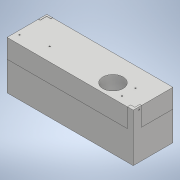
# Autodesk Inventor part: 2руб
Saved by Autodesk Inventor 2020 (Build 240168000, 168)
## iProperties
Created: 2020-02-01
Part Number: 2руб
Material: Типовые
Document SubType Name: Modeling
Designer: Css38
Density: 1 g/cm^3
Appearance: По умолчанию
Author: Css38
Autodesk Inventor part; units mm, degrees
ref_plane "YZ Plane" through (0, 0, 0) normal (1, 0, 0) x (0, 1, 0)
ref_plane "XZ Plane" through (0, 0, 0) normal (0, 1, 0) x (-1, 0, 0)
sketch "Эскиз1" plane through (0, 0, 0) normal (0, 0, 1) x (1, 0, 0)
  line L0 (-76.25, 24) -> (76.25, 24)
  line L1 (76.25, 24) -> (76.25, -24)
  line L2 (76.25, -24) -> (-76.25, -24)
  line L3 (-76.25, -24) -> (-76.25, 24)
  line L4 (-76.25, 24) -> (76.25, -24) construction
  line L5 (76.25, 24) -> (-76.25, -24) construction
  point P0 (0, 0)
  point P1 (0, 0)
  dimension "d35" = 152.5
  dimension "d36" = 48
  constraints: 12 end point, 2 parallel, 1 coincident, 1 horizontal, 1 midpoint, 1 perpendicular
  measures "d35" distance of L1.end L2.end
  measures "d36" distance of L2.end L0.start
extrude "Выдавливание1" add sketch "Эскиз1" along normal blind 30
sketch "Эскиз2" plane through (0, 0, 30) normal (0, 0, 1) x (1, 0, 0)
  line L0 (76.25, 24) -> (76.25, -24) construction
  line L1 (76.25, -24) -> (-76.25, -24) construction
  line L2 (-76.25, -24) -> (-76.25, 24) construction
  line L3 (-76.25, 24) -> (76.25, 24) construction
  line L4 (74.25, -20) -> (49.25, -20)
  line L5 (49.25, -20) -> (49.25, 5)
  line L6 (49.25, 5) -> (74.25, 5)
  line L7 (74.25, 5) -> (74.25, -20)
  point P0 (0, 0)
  dimension "d40" = 25
  dimension "d143" = 2
  dimension "d144" = 4
  constraints: 8 end point, 2 parallel, 2 perpendicular, 1 horizontal
  measures "d40" distance of L5.end L6.end
  measures "d143" distance between parallel lines of L0 L7
  measures "d144" distance between parallel lines of L1 L4
extrude "Выдавливание2" cut sketch "Эскиз2" against normal up to next
sketch "Эскиз3" plane through (0, 0, 30) normal (0, 0, 1) x (1, 0, 0)
  line L0 (49.25, 5) -> (49.25, -20)
  line L1 (49.25, -20) -> (74.25, -20)
  line L2 (74.25, -20) -> (74.25, 5)
  line L3 (74.25, 5) -> (49.25, 5)
  line L4 (76.25, 24) -> (76.25, -24) construction
  line L5 (76.25, -24) -> (-76.25, -24) construction
  line L6 (-76.25, 24) -> (76.25, 24) construction
  line L7 (76.25, 24) -> (-76.25, 24) projected
  line L8 (-76.25, 24) -> (76.25, 24)
  line L9 (76.25, 24) -> (76.25, -24)
  line L10 (76.25, -24) -> (-76.25, -24)
  line L11 (-76.25, 24) -> (-76.25, 22)
  line L12 (-76.25, 24) -> (-76.25, -24) construction
  line L13 (-76.25, 22) -> (1.25, 22)
  line L14 (1.25, 22) -> (1.25, 5)
  line L15 (1.25, 5) -> (21.25, 5)
  line L16 (21.25, 5) -> (21.25, -20)
  line L17 (21.25, -20) -> (-76.25, -20)
  line L18 (-76.25, -24) -> (-76.25, -20)
  line L19 (-76.25, -24) -> (76.25, -24) projected
  line L20 (76.25, -24) -> (76.25, 24) projected
  line L21 (74.25, -20) -> (49.25, -20) projected
  line L22 (49.25, -20) -> (49.25, 5) projected
  line L23 (49.25, 5) -> (74.25, 5) projected
  line L24 (74.25, 5) -> (74.25, -20) projected
  dimension "d50" = 2
  dimension "d63" = 28
  dimension "d130" = 20
  constraints: 34 end point, 13 collinear, 4 perpendicular, 2 parallel, 2 point on line
  measures "d50" distance of L6.start L11.end
  measures "d63" distance between parallel lines of L0 L16
  measures "d130" distance of L14.end L15.end
extrude "Выдавливание4" add sketch "Эскиз3" along normal blind 3
sketch "Эскиз4" plane through (0, 0, 33) normal (0, 0, 1) x (1, 0, 0)
  line L0 (49.25, 5) -> (49.25, -20) construction
  line L1 (49.25, -20) -> (74.25, -20) construction
  line L2 (74.25, -20) -> (74.25, 5) construction
  line L3 (74.25, 5) -> (49.25, 5) construction
  line L4 (76.25, 24) -> (76.25, -24) projected
  line L5 (76.25, -24) -> (-76.25, -24) projected
  line L6 (-76.25, -24) -> (-76.25, -20) projected
  line L7 (-76.25, -20) -> (21.25, -20) projected
  line L8 (21.25, -20) -> (21.25, 5) projected
  line L9 (21.25, 5) -> (1.25, 5) projected
  line L10 (1.25, 5) -> (1.25, 22) projected
  line L11 (1.25, 22) -> (-76.25, 22) projected
  line L12 (-76.25, 22) -> (-76.25, 24) projected
  line L13 (-76.25, 24) -> (76.25, 24) projected
  line L14 (21.25, -20) -> (21.25, 5) projected
  line L15 (21.25, 5) -> (49.25, 5) construction
  line L16 (49.25, 5) -> (49.25, -20) projected
  line L17 (49.25, -20) -> (21.25, -20) construction
  circle A0 centre (35.25, -7.5) radius 12.25
  line L18 (35.25, -7.5) -> (35.25, 5) construction
  line L19 (35.25, -7.5) -> (35.25, -20) construction
  line L20 (49.25, -20) -> (49.25, 5) construction
  line L21 (35.25, -7.5) -> (21.25, -7.5) construction
  line L22 (35.25, -7.5) -> (49.25, -7.5) construction
  point P0 (0, 0)
  dimension "d55" = 24.5
  constraints: 12 end point, 4 midpoint, 3 perpendicular, 2 collinear, 1 centre point, 1 point on line, 1 other
  measures "d55" diameter of A0
extrude "Выдавливание7" add sketch "Эскиз4" along normal blind 25
sketch "Эскиз6" plane through (21.25, -20, 30) normal (-1, 0, 0) x (0, 0, 1)
  line L0 (3, 0.25) -> (3, 24.75) construction
  line L1 (0, 25) -> (28, 25) projected
  line L2 (0, 0) -> (28, 0) projected
  line L3 (3, 25) -> (5.2, 25)
  line L4 (5.2, 25) -> (5.2, 0)
  line L5 (5.2, 0) -> (3, 0)
  line L6 (3, 0) -> (3, 25)
  point P0 (-30, 20)
  dimension "d66" = 2.2
  constraints: 8 end point, 2 parallel, 2 point on line, 1 collinear, 1 horizontal, 1 perpendicular
  measures "d66" distance of L4.end L5.end
extrude "Выдавливание8" cut sketch "Эскиз6" against normal up to surface (53 mm away) from surface at 0
sketch "Эскиз7" plane through (0, 0, 58) normal (0, 0, 1) x (1, 0, 0)
  line L0 (76.25, -24) -> (-76.25, -24) projected
  line L1 (-76.25, 24) -> (76.25, 24) projected
  line L2 (76.25, -24) -> (-76.25, -24)
  line L3 (-76.25, -24) -> (-76.25, 24)
  line L4 (-76.25, 24) -> (76.25, 24)
  line L5 (76.25, 24) -> (76.25, -24)
  circle A0 centre (35.25, -7.5) radius 12.25 projected
  point P0 (0, 0)
  constraints: 8 end point, 2 parallel, 1 horizontal, 1 perpendicular
extrude "Выдавливание9" add sketch "Эскиз7" against normal blind 17.15
ref_plane "РабПлоскость1" through (74.25, -20, 35.2) normal (0, 0, -1) x (-1, 0, 0)
split body "Разделение1" result two bodies by plane through (74.25, -20, 35.2) normal (0, 0, -1) first body at (-34.4167, 1.6667, 0.5)
sketch "Эскиз21" plane through (0, 0, 30) normal (0, 0, 1) x (1, 0, 0)
  line L0 (-76.25, -20) -> (21.25, -20) construction
  line L1 (21.25, -20) -> (21.25, 5) construction
  line L2 (21.25, 5) -> (1.25, 5) construction
  line L3 (1.25, 5) -> (1.25, 22) construction
  line L4 (1.25, 22) -> (-76.25, 22) construction
  line L5 (-76.25, -20) -> (-76.25, 22) construction
  line L6 (-76.25, -24) -> (-76.25, -20) construction
  line L7 (76.25, -24) -> (-76.25, -24) construction
  line L8 (76.25, 24) -> (76.25, -24) construction
  line L9 (-76.25, 24) -> (76.25, 24) construction
  line L10 (74.25, 5) -> (49.25, 5) construction
  line L11 (49.25, 5) -> (49.25, -20) construction
  line L12 (49.25, -20) -> (74.25, -20) construction
  line L13 (74.25, -20) -> (74.25, 5) construction
  line L14 (-76.25, -20) -> (-43.25, -20)
  line L15 (-43.25, -20) -> (-43.25, -7.5)
  line L16 (-43.25, -7.5) -> (-76.25, -7.5)
  line L17 (-76.25, -7.5) -> (-76.25, -20)
  line L18 (-76.25, 22) -> (-76.25, 24) projected
  point P0 (0, 0)
  dimension "d145" = 33
  dimension "d146" = 12.5
  constraints: 8 end point, 2 parallel, 1 horizontal, 1 perpendicular
  measures "d145" distance of L16.end L15.end
  measures "d146" distance of L15.end L14.end
extrude "Выдавливание26" cut sketch "Эскиз21" against normal blind 28 bodies 2
sketch "Эскиз22" plane through (0, 0, 2) normal (0, 0, 1) x (1, 0, 0)
  line L0 (-76.25, 24) -> (76.25, 24) construction
  line L1 (76.25, 24) -> (76.25, -24) construction
  line L2 (76.25, -24) -> (-76.25, -24) construction
  line L3 (-76.25, -24) -> (-76.25, -20) construction
  line L4 (-76.25, -20) -> (-76.25, -7.5) construction
  line L5 (-76.25, -7.5) -> (-76.25, 24) construction
  line L6 (-76.25, -20) -> (-43.25, -20) construction
  line L7 (-43.25, -20) -> (-43.25, -7.5) construction
  line L8 (-43.25, -7.5) -> (-76.25, -7.5) construction
  line L9 (74.25, 5) -> (49.25, 5) construction
  line L10 (49.25, 5) -> (49.25, -20) construction
  line L11 (49.25, -20) -> (74.25, -20) construction
  line L12 (74.25, -20) -> (74.25, 5) construction
  line L13 (-43.25, -7.5) -> (-47.75, -7.5)
  line L14 (-47.75, -7.5) -> (-47.75, -20)
  line L15 (-47.75, -20) -> (-43.25, -20)
  line L16 (-43.25, -20) -> (-43.25, -7.5)
  point P0 (0, 0)
  dimension "d149" = 4.5
  constraints: 8 end point, 2 parallel, 1 horizontal, 1 perpendicular, 1 point on line
  measures "d149" distance of L15.end L14.end
extrude "Выдавливание27" add sketch "Эскиз22" along normal blind 18 bodies 2
sketch "Эскиз23" plane through (0, 0, 20) normal (0, 0, 1) x (1, 0, 0)
  line L0 (-76.25, 24) -> (76.25, 24) construction
  line L1 (76.25, 24) -> (76.25, -24) construction
  line L2 (76.25, -24) -> (-76.25, -24) construction
  line L3 (-76.25, -24) -> (-76.25, -20) construction
  line L4 (-76.25, -20) -> (-47.75, -20) construction
  line L5 (-47.75, -20) -> (-47.75, -7.5) construction
  line L6 (-43.25, -7.5) -> (-47.75, -7.5) construction
  line L7 (-43.25, -20) -> (-43.25, -7.5) construction
  line L8 (-47.75, -20) -> (-43.25, -20) construction
  line L9 (-76.25, -7.5) -> (-76.25, 24) construction
  line L10 (-47.75, -7.5) -> (-76.25, -7.5) construction
  line L11 (74.25, 5) -> (49.25, 5) construction
  line L12 (49.25, 5) -> (49.25, -20) construction
  line L13 (49.25, -20) -> (74.25, -20) construction
  line L14 (74.25, -20) -> (74.25, 5) construction
  line L15 (-47.75, -20) -> (-43.25, -7.5) construction
  line L16 (-43.25, -20) -> (-47.75, -7.5) construction
  circle A0 centre (-45.5, -13.75) radius 0.75
  point P0 (0, 0)
  dimension "d152" = 1.5
  constraints: 4 end point, 1 centre point, 1 midpoint
  measures "d152" diameter of A0
extrude "Выдавливание28" cut sketch "Эскиз23" against normal blind 3 bodies 2
sketch "Эскиз24" plane through (0, 0, 30) normal (0, 0, 1) x (1, 0, 0)
  line L0 (-76.25, 24) -> (76.25, 24) construction
  line L1 (76.25, 24) -> (76.25, -24) construction
  line L2 (76.25, -24) -> (-76.25, -24) construction
  line L3 (-76.25, -24) -> (-76.25, -20) construction
  line L4 (-76.25, -20) -> (-43.25, -20) construction
  line L5 (-43.25, -20) -> (-43.25, -7.5) construction
  line L6 (-43.25, -7.5) -> (-76.25, -7.5) construction
  line L7 (-76.25, -7.5) -> (-76.25, 22) construction
  line L8 (1.25, 22) -> (-76.25, 22) construction
  line L9 (1.25, 5) -> (1.25, 22) construction
  line L10 (21.25, 5) -> (1.25, 5) construction
  line L11 (21.25, -20) -> (21.25, 5) construction
  line L12 (-43.25, -20) -> (21.25, -20) construction
  line L13 (74.25, 5) -> (49.25, 5) construction
  line L14 (49.25, 5) -> (49.25, -20) construction
  line L15 (49.25, -20) -> (74.25, -20) construction
  line L16 (74.25, -20) -> (74.25, 5) construction
  line L17 (-43.25, -7.5) -> (-43.25, -20) construction
  line L18 (-76.25, -20) -> (-76.25, -7.5) construction
  line L19 (-65.25, -13.75) -> (-48.2817, 16.8617)
  line L20 (-48.2817, 16.8617) -> (-27.533, -7.5)
  line L21 (-27.533, -7.5) -> (21.467, -7.5)
  line L22 (-76.25, 22) -> (-76.25, 24) projected
  point P0 (0, 0)
  point P1 (-43.25, -13.75)
  point P2 (49.25, -7.5)
  dimension "d155" = 11
  dimension "d156" = 49
  dimension "d157" = 35
  dimension "d161" = 32
  dimension "d162" = 61
  constraints: 6 end point, 2 midpoint, 1 horizontal, 1 horizontal alignment, 1 point on line
  measures "d155" distance from line of L18 L19.start
  measures "d156" distance of L20.end L21.end
  measures "d157" distance of L19.start L19.end
  measures "d161" distance of L19.end L20.end
  measures "d162" angle of L12 L19
sketch "Эскиз20" plane through (0, 0, 58) normal (0, 0, 1) x (1, 0, 0)
  line L0 (76.25, -24) -> (-76.25, -24) construction
  line L1 (-76.25, -24) -> (-76.25, 24) construction
  line L2 (59.5, -24) -> (-46, -24) construction
  line L3 (-46, -24) -> (-46, 8.5) construction
  line L4 (-46, 8.5) -> (59.5, 8.5) construction
  line L5 (0, -33.6) -> (0, 33.6) construction
  line L6 (59.5, 8.5) -> (59.5, -24) construction
  circle A0 centre (35.25, -7.5) radius 12.25 construction
  line L7 (-76.25, -24) -> (76.25, -24) construction
  line L8 (-76.25, -24) -> (76.25, -24) construction
  circle A1 centre (-71.25, -13.8) radius 0.5
  line L9 (-36, 8.5) -> (-36, -24) construction
  line L10 (49.5, -24) -> (49.5, 8.5) construction
  line L11 (-46, 8.5) -> (-36, -24) construction
  line L12 (-36, 8.5) -> (-46, -24) construction
  line L13 (59.5, 8.5) -> (49.5, -7.75) construction
  line L14 (49.5, -7.75) -> (59.5, -24) construction
  line L15 (49.5, -24) -> (59.5, -7.75) construction
  line L16 (59.5, -7.75) -> (49.5, 8.5) construction
  circle A2 centre (-41, -7.75) radius 0.5
  circle A3 centre (54.5, 0.375) radius 0.5
  circle A4 centre (54.5, -15.875) radius 0.5
  point P0 (0, 0)
  point P1 (-76.25, 14)
  dimension "d131" = 32.5
  dimension "d163" = 10.2
  dimension "d164" = 5
  dimension "d165" = 105.5
  dimension "d168" = 2
  dimension "d169" = 10
  dimension "d170" = 10
  dimension "d171" = 1
  constraints: 24 end point, 5 midpoint, 4 centre point, 4 point on line, 3 equal radius, 3 parallel, 3 perpendicular, 1 collinear, 1 horizontal
  measures "d131" distance of L2.end L3.end
  measures "d163" distance from line of L0 A1.centre
  measures "d164" distance from line of L1 A1.centre
  measures "d165" distance of L3.end L4.end
  measures "d168" distance edge to line of A0 L10
  measures "d169" distance between parallel lines of L6 L10
  measures "d170" distance between parallel lines of L3 L9
  measures "d171" diameter of A1
hole "Отверстие1" at (-71.25, -13.8, 58) at (-41, -7.75, 58) at (54.5, 0.375, 58) at (54.5, -15.875, 58) direction (0, 0, -1) diameter 1 depth 3 tip angle 118 countersink diameter 1.5 countersink angle 90 bodies 3
sketch "Эскиз25" plane through (0, 0, 30) normal (0, 0, 1) x (1, 0, 0)
  line L0 (-76.25, 24) -> (76.25, 24) construction
  line L1 (-76.25, 24) -> (-76.25, 14)
  line L2 (-76.25, -24) -> (-76.25, 24) construction
  line L3 (-76.25, 14) -> (-74.25, 14)
  line L4 (-76.25, -24) -> (-76.25, -20) construction
  line L5 (-76.25, -20) -> (-43.25, -20) construction
  line L6 (-43.25, -20) -> (-43.25, -7.5) construction
  line L7 (-43.25, -7.5) -> (-76.25, -7.5) construction
  line L8 (-76.25, -7.5) -> (-76.25, 22) construction
  line L9 (-76.25, 22) -> (-76.25, 24) construction
  line L10 (-76.25, 24) -> (76.25, 24) construction
  line L11 (76.25, 24) -> (76.25, -24) construction
  line L12 (76.25, -24) -> (-76.25, -24) construction
  line L13 (-43.25, -20) -> (21.25, -20) construction
  line L14 (21.25, -20) -> (21.25, 5) construction
  line L15 (21.25, 5) -> (1.25, 5) construction
  line L16 (1.25, 5) -> (1.25, 22) construction
  line L17 (1.25, 22) -> (-76.25, 22) construction
  line L18 (74.25, 5) -> (49.25, 5) construction
  line L19 (49.25, 5) -> (49.25, -20) construction
  line L20 (49.25, -20) -> (74.25, -20) construction
  line L21 (74.25, -20) -> (74.25, 5) construction
  line L22 (-74.25, 14) -> (-74.25, 22)
  line L23 (-74.25, 22) -> (-69.25, 22)
  line L24 (-69.25, 22) -> (-69.25, 24)
  line L25 (-69.25, 24) -> (-76.25, 24)
  line L26 (76.25, -24) -> (-76.25, -24) construction
  line L27 (76.25, -24) -> (76.25, -14)
  line L28 (76.25, 24) -> (76.25, -24) construction
  line L29 (76.25, -14) -> (74.25, -14)
  line L30 (74.25, -14) -> (74.25, -20)
  line L31 (74.25, -20) -> (69.25, -20)
  line L32 (69.25, -20) -> (69.25, -24)
  line L33 (69.25, -24) -> (76.25, -24)
  point P0 (0, 0)
  dimension "d179" = 10
  dimension "d180" = 2
  dimension "d181" = 5
  constraints: 24 end point, 7 point on line, 6 perpendicular, 3 horizontal, 2 parallel, 1 collinear
  measures "d179" distance of L0.start L1.end
  measures "d180" distance of L1.end L3.end
  measures "d181" distance of L22.end L23.end
extrude "Выдавливание29" add sketch "Эскиз25" along normal blind 28.1 bodies 2
sketch "Эскиз26" plane through (76.25, -24, 0) normal (1, 0, 0) x (0, 0, -1)
  line L0 (0, 4) -> (-58.1, 4) construction
  line L1 (-58.1, 10) -> (-58.1, 4) construction
  line L2 (-58.1, 10) -> (-52.1, 4) construction
  line L3 (-58.1, 4) -> (-52.1, 10) construction
  line L4 (-35.2, 10) -> (-58.1, 10) construction
  line L5 (-52.1, 4) -> (-52.1, 10) construction
  circle A0 centre (-55.1, 7) radius 0.5
  point P0 (0, 24)
  dimension "d184" = 1
  constraints: 6 end point, 2 perpendicular, 2 point on line, 1 centre point, 1 midpoint
  measures "d184" diameter of A0
hole "Отверстие2" at (76.25, -17, 55.1) direction (-1, 0, 0) diameter 1 end through all countersink diameter 1.5 countersink angle 90 bodies 2
sketch "Эскиз27" plane through (-76.25, -24, 0) normal (-1, 0, 0) x (0, 0, 1)
  line L0 (58.1, 46) -> (30, 46) construction
  line L1 (35.2, 46) -> (58.1, 46) construction
  line L2 (58.1, 46) -> (50.1, 38) construction
  line L3 (30, 38) -> (58.1, 38) construction
  line L4 (58.1, 38) -> (50.1, 46) construction
  line L5 (50.1, 46) -> (50.1, 38) construction
  circle A0 centre (54.1, 42) radius 0.5
  circle A1 centre (55.1, 7) radius 0.5 projected
  point P0 (0, 24)
  constraints: 6 end point, 2 perpendicular, 2 point on line, 1 centre point, 1 equal radius, 1 midpoint
hole "Отверстие3" at (-76.25, 18, 54.1) direction (1, 0, 0) diameter 1 end through all countersink diameter 1.5 countersink angle 90 bodies 2
sketch "Эскиз28" plane through (0, 0, 58) normal (0, 0, 1) x (1, 0, 0)
  line L0 (74.25, -14) -> (76.25, -14) construction
  line L1 (76.25, -14) -> (76.25, -24) construction
  line L2 (76.25, -24) -> (69.25, -24) construction
  line L3 (69.25, -24) -> (69.25, -20) construction
  line L4 (69.25, -20) -> (74.25, -20) construction
  line L5 (74.25, -20) -> (74.25, -14) construction
  line L6 (-74.25, 22) -> (-74.25, 14) construction
  line L7 (-74.25, 14) -> (-76.25, 14) construction
  line L8 (-76.25, 14) -> (-76.25, 24) construction
  line L9 (-76.25, 24) -> (-69.25, 24) construction
  line L10 (-69.25, 24) -> (-69.25, 22) construction
  line L11 (-69.25, 22) -> (-74.25, 22) construction
  circle A0 centre (54.5, 0.375) radius 0.75 construction
  circle A1 centre (-71.25, -13.8) radius 0.75 construction
  circle A2 centre (-41, -7.75) radius 0.75 construction
  circle A3 centre (54.5, -15.875) radius 0.75 construction
  line L12 (-76.25, -24) -> (-76.25, 24) construction
  line L13 (-76.25, 24) -> (76.25, 24) construction
  line L14 (76.25, 24) -> (76.25, -24) construction
  line L15 (76.25, -24) -> (-76.25, -24) construction
  circle A4 centre (35.25, -7.5) radius 12.25 construction
  line L16 (-74.15, 13.9) -> (-74.15, 21.9)
  line L17 (-74.15, 21.9) -> (-69.15, 21.9)
  line L18 (-69.15, 21.9) -> (-69.15, 24.1)
  line L19 (-69.15, 24.1) -> (-76.35, 24.1)
  line L20 (-76.35, 24.1) -> (-76.35, 13.9)
  line L21 (-76.35, 13.9) -> (-74.15, 13.9)
  line L22 (74.15, -19.9) -> (69.15, -19.9)
  line L23 (69.15, -19.9) -> (69.15, -24.1)
  line L24 (69.15, -24.1) -> (76.35, -24.1)
  line L25 (76.35, -24.1) -> (76.35, -13.9)
  line L26 (76.35, -13.9) -> (74.15, -13.9)
  line L27 (74.15, -13.9) -> (74.15, -19.9)
  point P0 (0, 0)
  dimension "d199" = 0.1
  dimension "d200" = 0.1
  constraints: 24 end point, 10 other
  measures "d199" distance between parallel lines of L6 L16
  measures "d200" distance between parallel lines of L4 L22
extrude "Выдавливание30" cut sketch "Эскиз28" against normal through all bodies 3
sketch "Эскиз29" plane through (74.15, -19.9, 58) normal (1, 0, 0) x (0, 0, -1)
  circle A0 centre (2.9, 2.9) radius 0.5 construction
  circle A1 centre (3, 2.9) radius 0.5
  point P0 (58, 19.9)
  dimension "d203" = 0.1
  constraints: 1 centre point, 1 equal radius, 1 horizontal alignment
  measures "d203" distance of A0.centre A1.centre
hole "Отверстие4" at (74.15, -17, 55) direction (-1, 0, 0) diameter 1 depth 4 tip angle 118 countersink diameter 1.5 countersink angle 90 bodies 3
sketch "Эскиз30" plane through (-74.15, 13.9, 58) normal (-1, 0, 0) x (0, 0, 1)
  circle A0 centre (-3.9, 4.1) radius 0.5 construction
  circle A1 centre (-4, 4.1) radius 0.5
  point P0 (-58, -13.9)
  dimension "d211" = 0.1
  constraints: 1 centre point, 1 equal radius, 1 horizontal alignment
  measures "d211" distance of A0.centre A1.centre
hole "Отверстие5" at (-74.15, 18, 54) direction (1, 0, 0) diameter 1 depth 4 tip angle 118 countersink diameter 1.5 countersink angle 90 bodies 3
